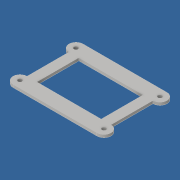
# Autodesk Inventor part: templateMount
Saved by Autodesk Inventor 2016 (Build 200138000, 138)
## iProperties
Created: 2017-06-20
Part Number: templateMount
Material: Generisch
Document SubType Name: Modeling
Designer: 4ndreas
Density: 1 g/cm^3
Appearance: Vorgabe
Author: 4ndreas
Autodesk Inventor part; units mm, degrees
ref_plane "YZ Plane" through (0, 0, 0) normal (1, 0, 0) x (0, 1, 0)
ref_plane "XZ Plane" through (0, 0, 0) normal (0, 1, 0) x (-1, 0, 0)
ref_plane "XY Plane" through (0, 0, 0) normal (0, 0, 1) x (1, 0, 0)
sketch "Skizze1" plane through (0, 0, 0) normal (0, 0, 1) x (1, 0, 0)
  line L0 (-30, -20) -> (30, -20)
  line L1 (30, -20) -> (30, 20)
  line L2 (30, 20) -> (-30, 20)
  line L3 (-30, 20) -> (-30, -20)
  line L4 (-30, -20) -> (30, 20) construction
  line L5 (30, -20) -> (-30, 20) construction
  circle A0 centre (-30, 20) radius 5
  circle A1 centre (-30, -20) radius 5
  circle A2 centre (30, -20) radius 5
  circle A3 centre (30, 20) radius 5
  line L6 (-30, 25) -> (30, 25)
  line L7 (30, 25) -> (30, 15)
  line L8 (30, 15) -> (-30, 15)
  line L9 (-30, 15) -> (-30, 25)
  line L10 (-30, -15) -> (30, -15)
  line L11 (30, -15) -> (30, -25)
  line L12 (30, -25) -> (-30, -25)
  line L13 (-30, -25) -> (-30, -15)
  line L14 (-23, 15) -> (23, 15)
  line L15 (23, 15) -> (23, -15)
  line L16 (23, -15) -> (-23, -15)
  line L17 (-23, -15) -> (-23, 15)
  point P0 (0, 0)
  dimension "d0" = 40
  dimension "d1" = 60
  dimension "d2" = 7
  dimension "d3" = 10
  dimension "d4" = 7
  constraints: 36 end point, 8 parallel, 5 point on line, 4 coincident, 4 horizontal, 4 perpendicular, 4 point on circle, 3 midpoint, 2 centre point, 2 vertical alignment, 5 other
  measures "d0" distance between parallel lines of L0 L2
  measures "d1" distance between parallel lines of L1 L3
  measures "d2" distance between parallel lines of L3 L17
  measures "d3" diameter of A0
  measures "d4" distance between parallel lines of L15 L1
extrude "Extrusion1" add sketch "Skizze1" along normal blind 2 contours L3 A1 L0 | L13 A1 L3 | L0 A1 L13 | A1 L10 A2 L0 | L0 A2 L12 A1 | L3 L8 L17 L10 | A2 L1 L0 | L0 L11 A2 | A0 L9 L3 | L3 L2 A0 | A0 L2 A3 L8 | L11 L1 A2 | L10 L15 L8 L1 | L9 A0 L2 | L6 A3 L2 A0 | A3 L2 L1 | L1 L7 A3 | L7 L2 A3
sketch "Skizze2" plane through (0, 0, 2) normal (0, 0, 1) x (1, 0, 0)
  line L0 (23, -15) -> (-23, -15) projected
  line L1 (-23, -15) -> (-23, 15) projected
  line L2 (-23, 15) -> (23, 15) projected
  line L3 (23, 15) -> (23, -15) projected
  line L4 (30, -15) -> (30, 15) projected
  arc A0 (30, 15) -> (30, 25) centre (30, 20) ccw projected
  line L5 (30, 25) -> (-30, 25) projected
  arc A1 (-30, 25) -> (-30, 15) centre (-30, 20) ccw projected
  line L6 (-30, 15) -> (-30, -15) projected
  arc A2 (-30, -15) -> (-30, -25) centre (-30, -20) ccw projected
  line L7 (-30, -25) -> (30, -25) projected
  arc A3 (30, -25) -> (30, -15) centre (30, -20) ccw projected
  point P0 (0, 0)
hole "Bohrung1" at (-30, 20, 2) at (-30, -20, 2) at (30, -20, 2) at (30, 20, 2) direction (0, 0, -1) diameter 3 end through all
equation "\"d4\" = d2"
